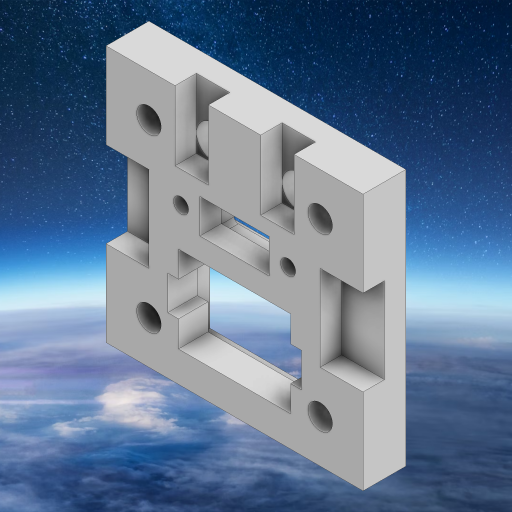
# Autodesk Inventor part: power_signal_socket_fixed
Saved by Autodesk Inventor 2023 (Build 270158000, 158)
## iProperties
Created: 2023-10-30
Part Number: power_signal_socket_fixed
Material: 一般
Document SubType Name: Modeling
Designer: 310611102
Density: 1 g/cm^3
Appearance: 預設
Author: 310611102
Autodesk Inventor part; units mm, degrees
ref_plane "YZ Plane" through (0, 0, 0) normal (1, 0, 0) x (0, 1, 0)
ref_plane "XZ Plane" through (0, 0, 0) normal (0, 1, 0) x (-1, 0, 0)
ref_plane "XY Plane" through (0, 0, 0) normal (0, 0, 1) x (1, 0, 0)
sketch "Sketch1" plane through (0, 0, 0) normal (0, 0, 1) x (1, 0, 0)
  line L0 (-30, 30) -> (30, 30)
  line L1 (30, 30) -> (30, -30)
  line L2 (30, -30) -> (-30, -30)
  line L3 (-30, -30) -> (-30, 30)
  line L4 (-30, 30) -> (30, -30) construction
  line L5 (30, 30) -> (-30, -30) construction
  line L6 (0, 0) -> (0, -32.9158)
  circle A0 centre (-12.5, 6.5) radius 1.75
  circle A1 centre (12.5, 6.5) radius 1.75
  line L7 (-8.1, 10.5) -> (8.1, 10.5)
  line L8 (8.1, 10.5) -> (8.1, 2.5)
  line L9 (8.1, 2.5) -> (-8.1, 2.5)
  line L10 (-8.1, 2.5) -> (-8.1, 10.5)
  line L11 (-8.1, 10.5) -> (8.1, 2.5) construction
  line L12 (8.1, 10.5) -> (-8.1, 2.5) construction
  line L13 (13.1, -2.65) -> (-13.1, -2.65)
  line L14 (-13.1, -2.65) -> (-13.1, -22.85)
  line L15 (-13.1, -22.85) -> (13.1, -22.85)
  line L16 (13.1, -22.85) -> (13.1, -2.65)
  line L17 (13.1, -2.65) -> (-13.1, -22.85) construction
  line L18 (-13.1, -2.65) -> (13.1, -22.85) construction
  line L19 (8.9501, 0.5324) -> (10, 12.5324)
  line L20 (-8.9501, 0.5324) -> (-10, 12.5324)
  line L21 (10, 12.5324) -> (-10, 12.5324)
  line L22 (-8.9501, 0.5324) -> (8.9501, 0.5324)
  line L23 (10, 12.5324) -> (-8.9501, 0.5324)
  line L24 (-10, 12.5324) -> (8.9501, 0.5324)
  line L25 (13.1, -16.75) -> (15.6, -16.75)
  line L26 (15.6, -16.75) -> (15.6, -8.75)
  line L27 (15.6, -8.75) -> (13.1, -8.75)
  line L28 (13.1, -8.75) -> (13.1, -16.75)
  line L29 (-13.1, -8.75) -> (-15.6, -8.75)
  line L30 (-15.6, -8.75) -> (-15.6, -16.75)
  line L31 (-15.6, -16.75) -> (-13.1, -16.75)
  line L32 (-13.1, -16.75) -> (-13.1, -8.75)
  line L33 (0, -12.75) -> (7.7881, -12.75)
  point P0 (0, 6.5)
  point P1 (0, 6.2)
  dimension "d0" = 60
  dimension "d1" = 60
  dimension "d10" = 3.5
  dimension "d11" = 3.5
  dimension "d12" = 25
  dimension "d15" = 16.2
  dimension "d16" = 8
  dimension "d21" = 26.2
  dimension "d22" = 20.2
  dimension "d32" = 17.25
  dimension "d33" = 19.25
  dimension "d61" = 5
  dimension "d62" = 20
  dimension "d63" = 12
  dimension "d67" = 0.3
  dimension "d68" = 2.5
  dimension "d69" = 8
  constraints: 68 end point, 11 parallel, 7 horizontal, 6 midpoint, 5 perpendicular, 5 point on line, 2 centre point, 2 collinear, 2 equal length, 1 horizontal alignment, 1 symmetric about line, 1 vertical, 3 other
  measures "d0" distance of L0.start L0.end
  measures "d1" distance of L0.end L1.end
  measures "d10" diameter of A0
  measures "d11" diameter of A1
  measures "d12" distance of A1.centre A0.centre
  measures "d15" distance of L7.start L7.end
  measures "d16" distance of L9.end L7.start
  measures "d21" distance of L13.start L13.end
  measures "d22" distance of L13.end L14.end
  measures "d32" distance from line of L2 L33.start
  measures "d33" distance of L33.start point (0, 6.5)
  measures "d61" angle of L8 L19
  measures "d62" distance of L20.end L19.end
  measures "d63" distance between parallel lines of L22 L21
  measures "d67" distance of point (0, 6.5) point (0, 6.2)
  measures "d68" distance of L26.end L27.end
  measures "d69" distance of L29.end L30.end
extrude "Extrusion1" add sketch "Sketch1" along normal blind 10 contours L0 L1 L2 L3 | L10 L9 L23 L20 L24 L7 | L24 L21 L23 L7 | L23 L19 L24 L9 L8 L7 | L9 L24 L22 L23
extrude "Extrusion10" cut sketch "Sketch1" along normal blind 5 contours L10 L9 L23 L20 L24 L7 | L24 L21 L23 L7 | L23 L19 L24 L9 L8 L7 | L9 L24 L22 L23
fillet "Fillet1" radius 1 4 edges at (10, 12.5324, 2.5) (-10, 12.5324, 2.5) (-8.9501, 0.5324, 2.5) (8.9501, 0.5324, 2.5)
sketch "Sketch2" plane through (0, 0, 0) normal (0, 0, -1) x (-1, 0, 0)
  line L0 (-15.75, -0.5) -> (15.75, -0.5)
  line L1 (15.75, -0.5) -> (15.75, -25)
  line L2 (15.75, -25) -> (-15.75, -25)
  line L3 (-15.75, -25) -> (-15.75, -0.5)
  line L4 (-15.75, -0.5) -> (15.75, -25) construction
  line L5 (15.75, -0.5) -> (-15.75, -25) construction
  line L6 (13.1, -22.85) -> (13.1, -2.65) projected
  point P0 (0, 0)
  point P1 (0, -12.75)
  point P2 (-15.75, -12.75)
  point P3 (13.1, -12.75)
  dimension "d17" = 31.5
  dimension "d18" = 24.5
  constraints: 12 end point, 4 midpoint, 2 horizontal alignment, 2 parallel, 1 horizontal, 1 perpendicular, 1 vertical alignment
  measures "d17" distance of L0.start L0.end
  measures "d18" distance of L0.end L1.end
extrude "Extrusion2" cut sketch "Sketch2" against normal blind 3.1
sketch "Sketch3" plane through (0, 0, 0) normal (0, 0, -1) x (-1, 0, 0)
  line L0 (-15.5, 13.1) -> (15.5, 13.1)
  line L1 (15.5, 13.1) -> (15.5, -0.1)
  line L2 (15.5, -0.1) -> (-15.5, -0.1)
  line L3 (-15.5, -0.1) -> (-15.5, 13.1)
  line L4 (-15.5, 13.1) -> (15.5, -0.1) construction
  line L5 (15.5, 13.1) -> (-15.5, -0.1) construction
  circle A0 centre (-12.5, 6.5) radius 1.75 projected
  point P0 (0, 0)
  point P1 (0, 6.5)
  dimension "d23" = 31
  dimension "d24" = 13.2
  constraints: 12 end point, 2 midpoint, 2 parallel, 1 horizontal, 1 horizontal alignment, 1 perpendicular, 1 vertical alignment
  measures "d23" distance of L0.start L0.end
  measures "d24" distance of L0.end L1.end
extrude "Extrusion3" cut sketch "Sketch3" against normal blind 1.1 contours L0 L1 L2 L3 | A0
sketch "Sketch4" plane through (0, 0, 0) normal (0, 0, -1) x (-1, 0, 0)
  circle A0 centre (-12.5, 6.5) radius 1.75 projected
  line L0 (-9.65, 8.1454) -> (-9.65, 4.8546)
  line L1 (-9.65, 4.8546) -> (-12.5, 3.2091)
  line L2 (-12.5, 3.2091) -> (-15.35, 4.8546)
  line L3 (-15.35, 4.8546) -> (-15.35, 8.1454)
  line L4 (-15.35, 8.1454) -> (-12.5, 9.7909)
  line L5 (-12.5, 9.7909) -> (-9.65, 8.1454)
  circle A1 centre (12.5, 6.5) radius 1.75 projected
  line L6 (12.5, 9.7909) -> (15.35, 8.1454)
  line L7 (15.35, 8.1454) -> (15.35, 4.8546)
  line L8 (15.35, 4.8546) -> (12.5, 3.2091)
  line L9 (12.5, 3.2091) -> (9.65, 4.8546)
  line L10 (9.65, 4.8546) -> (9.65, 8.1454)
  line L11 (9.65, 8.1454) -> (12.5, 9.7909)
  point P0 (0, 0)
  point P1 (-9.65, 6.5)
  point P2 (-15.35, 6.5)
  dimension "d27" = 5.7
  dimension "d30" = 5.7
  constraints: 24 end point, 2 coincident, 2 midpoint, 2 vertical alignment, 26 other
  measures "d27" distance of point (-9.65, 6.5) point (-15.35, 6.5)
  measures "d30" distance between parallel lines of L7 L10
extrude "Extrusion4" cut sketch "Sketch4" against normal blind 3.6 contours A0 | L0 L1 L2 L3 L4 L5 | A1 | L6 L7 L8 L9 L10 L11
sketch "Sketch5" plane through (0, 0, 10) normal (0, 0, 1) x (1, 0, 0)
  circle A0 centre (-20, 20) radius 2.85
  line L0 (0, 0) -> (0, 27.5529)
  line L1 (0, 0) -> (35.0302, 0)
  circle A1 centre (20, 20) radius 2.85
  circle A2 centre (-20, -20) radius 2.85
  circle A3 centre (20, -20) radius 2.85
  dimension "d34" = 5.7
  dimension "d35" = 40
  dimension "d36" = 40
  constraints: 4 centre point, 4 end point, 3 symmetric about line, 1 horizontal, 1 vertical, 3 other
  measures "d34" diameter of A0
  measures "d35" diameter of A0.centre L0
  measures "d36" diameter of A0.centre L1
extrude "Extrusion5" cut sketch "Sketch5" against normal blind 4
sketch "Sketch6" plane through (0, 0, 0) normal (0, 0, -1) x (-1, 0, 0)
  circle A0 centre (-10, 18) radius 3.9
  circle A1 centre (10, 18) radius 3.9
  line L0 (30, -30) -> (-30, -30) projected
  line L1 (0, 0) -> (0, 19.7)
  dimension "d39" = 7.8
  dimension "d40" = 7.8
  dimension "d41" = 48
  dimension "d42" = 20
  constraints: 2 centre point, 2 end point, 1 horizontal alignment, 1 symmetric about line, 1 vertical
  measures "d39" diameter of A0
  measures "d40" diameter of A1
  measures "d41" distance from line of L0 A1.centre
  measures "d42" distance of A1.centre A0.centre
extrude "Extrusion6" cut sketch "Sketch6" against normal through all
sketch "Sketch8" plane through (0, 0, 10) normal (0, 0, 1) x (1, 0, 0)
  line L0 (-13.9, 30) -> (-6.1, 30)
  line L1 (-6.1, 30) -> (-6.1, 13.8)
  line L2 (-6.1, 13.8) -> (-13.9, 13.8)
  line L3 (-13.9, 13.8) -> (-13.9, 30)
  line L4 (0, 0) -> (0, 35.6896)
  line L5 (13.9, 30) -> (6.1, 30)
  line L6 (6.1, 30) -> (6.1, 13.8)
  line L7 (6.1, 13.8) -> (13.9, 13.8)
  line L8 (13.9, 13.8) -> (13.9, 30)
  circle A0 centre (-10, 18) radius 3.9 projected
  line L9 (-10, 18) -> (-10, 21.5524)
  line L10 (30, 30) -> (-30, 30) projected
  dimension "d46" = 7.8
  dimension "d48" = 4.2
  constraints: 20 end point, 4 symmetric about line, 2 parallel, 2 vertical, 1 collinear, 1 horizontal, 1 perpendicular, 1 other
  measures "d46" distance of L0.start L0.end
  measures "d48" distance from line of L2 L9.start
extrude "Extrusion7" cut sketch "Sketch8" against normal blind 5 contours L5 L8 L7 L6 | L0 L1 A0 L3 | A0 L1 L2 L3
sketch "Sketch9" plane through (-20, 20, 6) normal (0, 0, 1) x (1, 0, 0)
  circle A0 centre (0, 0) radius 1.75
  circle A1 centre (40, 0) radius 2.85 projected
  circle A2 centre (40, 0) radius 1.75
  circle A3 centre (0, -40) radius 2.85 projected
  circle A4 centre (0, -40) radius 1.75
  circle A5 centre (40, -40) radius 2.85 projected
  circle A6 centre (40, -40) radius 1.75
  point P0 (20, -20)
  dimension "d51" = 3.5
  dimension "d52" = 3.5
  dimension "d53" = 3.5
  dimension "d54" = 3.5
  constraints: 4 centre point, 3 coincident
  measures "d51" diameter of A0
  measures "d52" diameter of A2
  measures "d53" diameter of A4
  measures "d54" diameter of A6
extrude "Extrusion8" cut sketch "Sketch9" against normal through all contours A0 | A2 | A4 | A6
sketch "Sketch10" plane through (0, 0, 10) normal (0, 0, 1) x (1, 0, 0)
  line L0 (-30, 30) -> (-30, -30) projected
  line L1 (-20, 10) -> (-30, 10)
  line L2 (-30, 10) -> (-30, -10)
  line L3 (-30, -10) -> (-20, -10)
  line L4 (-20, -10) -> (-20, 10)
  line L5 (-20, 10) -> (-30, -10) construction
  line L6 (-30, 10) -> (-20, -10) construction
  line L7 (0, 0) -> (0, 15.7555)
  line L8 (20, 10) -> (30, 10)
  line L9 (30, 10) -> (30, -10)
  line L10 (30, -10) -> (20, -10)
  line L11 (20, -10) -> (20, 10)
  line L12 (20, 10) -> (30, -10) construction
  line L13 (30, 10) -> (20, -10) construction
  point P0 (-25, 0)
  point P1 (25, 0)
  dimension "d57" = 20
  dimension "d58" = 10
  constraints: 26 end point, 5 symmetric about line, 2 midpoint, 2 parallel, 1 horizontal, 1 horizontal alignment, 1 perpendicular, 1 point on line, 1 vertical
  measures "d57" distance of L3.end L1.start
  measures "d58" distance of L1.start L1.end
extrude "Extrusion9" cut sketch "Sketch10" against normal blind 5
equation "\"d10\" = d2"
equation "\"d11\" = d2"
equation "\"d30\" = d27"
equation "\"d39\" = d40"
equation "\"d52\" = d51"
equation "\"d53\" = d51"
equation "\"d54\" = d51"
equation "\"d2\" = 3.5"
body "Solid1"
